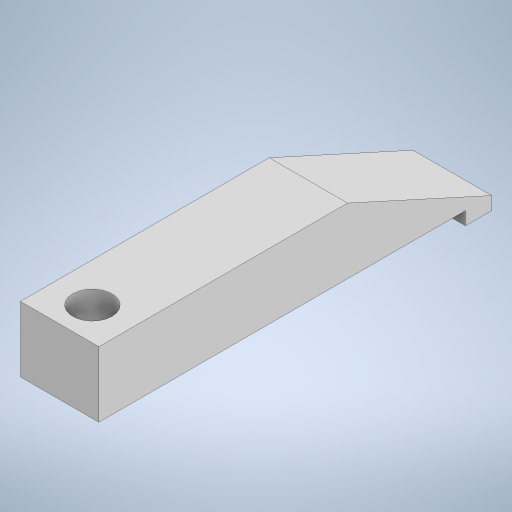
# Autodesk Inventor part: Soporte PCB pieza plastico
Saved by Autodesk Inventor 2023 (Build 270158000, 158)
## iProperties
Created: 2023-02-26
Part Number: Soporte PCB pieza plastico
Material: Genérico
Document SubType Name: Modeling
Designer: sergi
Density: 1 g/cm^3
Appearance: Valor por defecto
Author: sergi
Autodesk Inventor part; units mm, degrees
ref_plane "YZ Plane" through (0, 0, 0) normal (1, 0, 0) x (0, 1, 0)
ref_plane "XZ Plane" through (0, 0, 0) normal (0, 1, 0) x (-1, 0, 0)
ref_plane "XY Plane" through (0, 0, 0) normal (0, 0, 1) x (1, 0, 0)
sketch "Boceto1" plane through (0, 0, 0) normal (0, 1, 0) x (-1, 0, 0)
  line L0 (-3, -15) -> (3, -15)
  line L1 (3, -15) -> (3, 15)
  line L2 (3, 15) -> (-3, 15)
  line L3 (-3, 15) -> (-3, -15)
  line L4 (-3, -15) -> (3, 15) construction
  line L5 (3, -15) -> (-3, 15) construction
  circle A0 centre (0, 12.5) radius 1.5
  point P0 (0, 0)
  point P1 (0, 15)
  dimension "d0" = 6
  dimension "d1" = 30
  dimension "d3" = 3
  dimension "d12" = 2.5
  constraints: 12 end point, 3 midpoint, 2 parallel, 1 centre point, 1 horizontal, 1 perpendicular
  measures "d0" distance of L2.end L1.end
  measures "d1" distance of L1.end L0.end
  measures "d3" diameter of A0
  measures "d12" distance of point (0, 15) A0.centre
extrude "Extrusión1" add sketch "Boceto1" along normal blind 5
chamfer "Chaflán1" distance 11 distance2 5 1 edges at (0, 5, -15) measured on face at (-0.0603, 5, -6.3297)
sketch "Boceto2" plane through (0, 0, 0) normal (0, -1, 0) x (1, 0, 0)
  line L0 (3, 15) -> (3, -15) projected
  line L1 (-3, -15) -> (-3, 15) projected
  line L2 (3, -15) -> (-3, -15)
  line L3 (-3, -15) -> (-3, -13)
  line L4 (-3, -13) -> (3, -13)
  line L5 (3, -13) -> (3, -15)
  point P0 (0, 0)
  point P1 (-3, -15)
  point P2 (3, -13)
  dimension "d9" = 2
  constraints: 8 end point, 2 parallel, 1 horizontal, 1 perpendicular, 1 point on line
  measures "d9" distance of L2.end L3.end
extrude "Extrusión2" add sketch "Boceto2" along normal blind 1
